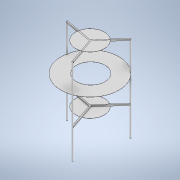
# Autodesk Inventor part: boiler_plates
Saved by Autodesk Inventor 2020 (Build 240168000, 168)
## iProperties
Created: 2022-08-31
Part Number: boiler_plates
Material: Generic
Document SubType Name: Modeling
Designer: Intuito_PC
Density: 1 g/cm^3
Appearance: Default
Author: Intuito_PC
Autodesk Inventor part; units mm, degrees
ref_plane "YZ Plane" through (0, 0, 0) normal (1, 0, 0) x (0, 1, 0)
ref_plane "XZ Plane" through (0, 0, 0) normal (0, 1, 0) x (-1, 0, 0)
sketch "Sketch1" plane through (0, 0, 0) normal (0, 1, 0) x (-1, 0, 0)
  circle A0 centre (-83.0821, 235.7909) radius 5
  circle A1 centre (-162.6599, -189.8467) radius 5
  circle A2 centre (245.742, -45.9443) radius 5
  point P0 (0, 0)
  dimension "d3" = 10
  dimension "d4" = 10
  dimension "d5" = 10
  constraints: 3 centre point
  measures "d3" diameter of A0
  measures "d4" diameter of A1
  measures "d5" diameter of A2
extrude "Extrusion1" add sketch "Sketch1" along normal blind 750
sketch "Sketch2" plane through (83.0821, 750, 235.7909) normal (0, 1, 0) x (1, 0, 0)
  circle A0 centre (-328.8241, 281.7352) radius 5 projected
  circle A1 centre (79.5778, 425.6376) radius 5 projected
  line L0 (-326.9753, 276.3685) -> (-84.2277, 230.0921)
  line L1 (-82.7079, 228.7691) -> (-5.5677, 1.0437)
  circle A2 centre (0, 0) radius 5 projected
  line L2 (-325.1511, 286.0493) -> (-86.7137, 240.5946)
  line L3 (-86.7137, 240.5946) -> (74.0056, 426.7207)
  line L4 (81.481, 420.2957) -> (-74.7837, 239.3284)
  line L5 (-75.1642, 237.3796) -> (3.7927, 4.2915)
  arc A3 (-327.4871, 284.4754) -> (-328.5709, 278.6773) centre (-83.0821, 235.7909) ccw
  arc A4 (-3.0309, -0.2086) -> (2.5859, 1.7717) centre (-83.0821, 235.7909) ccw
  arc A5 (81.2864, 423.1061) -> (76.8025, 426.9477) centre (-83.0821, 235.7909) ccw
  arc A6 (-82.7079, 228.7691) -> (-84.2277, 230.0921) centre (-84.6022, 228.1275) ccw
  arc A7 (76.8025, 426.9477) -> (74.0056, 426.7207) centre (75.5193, 425.4136) ccw
  arc A8 (81.481, 420.2957) -> (81.2864, 423.1061) centre (79.9673, 421.6028) ccw
  arc A9 (2.5859, 1.7717) -> (3.7927, 4.2915) centre (1.8984, 3.6499) ccw
  arc A10 (-5.5677, 1.0437) -> (-3.0309, -0.2086) centre (-3.6734, 1.6854) ccw
  arc A11 (-74.7837, 239.3284) -> (-75.1642, 237.3796) centre (-73.2699, 238.0212) ccw
  arc A12 (-328.5709, 278.6773) -> (-326.9753, 276.3685) centre (-326.6007, 278.3331) ccw
  arc A13 (-325.1511, 286.0493) -> (-327.4871, 284.4754) centre (-325.5257, 284.0846) ccw
  point P0 (-83.0821, 235.7909)
  point P1 (-328.9022, 276.7358)
  point P2 (-4.9283, -0.8437)
  point P3 (75.2872, 428.2049)
  point P4 (82.7726, 421.7915)
  point P5 (-75.5311, 238.4628)
  point P6 (4.4165, 2.45)
  dimension "d8" = 2
  dimension "d9" = 2
  constraints: 29 point on circle, 16 tangent, 12 end point, 11 centre point, 9 point on line, 6 equal radius, 3 parallel, 4 other
  measures "d8" radius of A6
  measures "d9" radius of A12
extrude "Extrusion2" add sketch "Sketch2" against normal blind 10 contours A0 A12 A3 A13 | A0 A13 L2 L3 A7 A1 A8 L4 A11 L5 A9 A2 A10 L1 A6 L0 A12 | A7 A5 A8 A1 | A2 A9 A4 A10 picked at (-326.6818, 281.2494) picked at (78.1424, 423.9745) picked at (-0.6818, 2.0889)
ref_plane "Work Plane1" through (0, 500, 0) normal (0, 1, 0) x (1, 0, 0)
mirror "Mirror1" about plane through (0, 500, 0) normal (0, 1, 0) of "Extrusion2"
sketch "Sketch3" plane through (0, 750, 0) normal (0, 1, 0) x (1, 0, 0)
  circle A0 centre (0, 0) radius 125
  dimension "d13" = 250
  constraints: 1 centre point, 1 coincident
  measures "d13" diameter of A0
extrude "Extrusion3" add sketch "Sketch3" along normal blind 1
mirror "Mirror2" about plane through (0, 500, 0) normal (0, 1, 0) of "Extrusion3"
sketch "Sketch4" plane through (0, 500, 0) normal (0, 1, 0) x (1, 0, 0)
  circle A0 centre (0, 0) radius 252.3793
  circle A1 centre (0, 0) radius 125
  constraints: 2 centre point, 2 coincident
extrude "Extrusion5" add sketch "Sketch4" along normal blind 1 contours A0 | A1
sketch "Sketch5" plane through (0, 501, 0) normal (0, 1, 0) x (1, 0, 0)
  circle A0 centre (3.3929, 3.4645) radius 124.3815
  point P0 (0, 0)
  constraints: 1 centre point
extrude "Extrusion6" cut sketch "Sketch5" against normal blind 1
body "Solid1"
